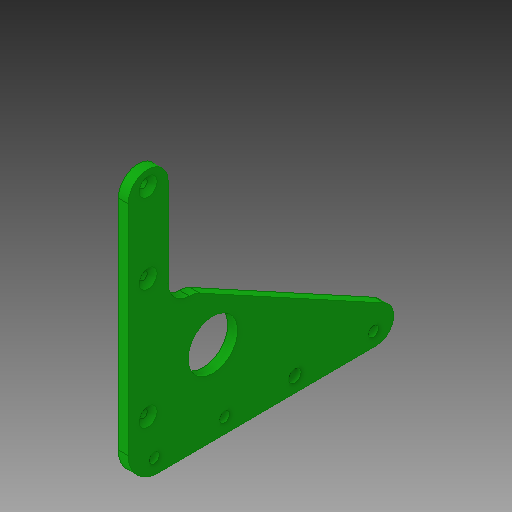
# Autodesk Inventor part: support plate
Saved by Autodesk Inventor 2017 SP1 (Build 210196100, 196)
## iProperties
Created: 2018-01-20
Part Number: support plate
Material: Aluminum 6061
Document SubType Name: Modeling
Designer: Ben
Density: 2.7 g/cm^3
Appearance: Dark Green
Mass: 193.553 g
Surface Area: 279.348 cm^2
Volume: 71.6862 cm^3
Author: Ben
Autodesk Inventor part; units mm, degrees
ref_plane "YZ Plane" through (0, 0, 0) normal (1, 0, 0) x (0, 1, 0)
ref_plane "XZ Plane" through (0, 0, 0) normal (0, 1, 0) x (-1, 0, 0)
ref_plane "XY Plane" through (0, 0, 0) normal (0, 0, 1) x (1, 0, 0)
sketch "Sketch1" plane through (0, 0, 0) normal (1, 0, 0) x (0, 1, 0)
  circle A0 centre (0, 0) radius 2.667
  circle A1 centre (76.2, 0) radius 2.667
  circle A2 centre (127, 0) radius 2.667
  line L0 (127, 0) -> (0, 0) construction
  line L1 (-15.2262, 12.7) -> (123.825, 12.7)
  line L2 (123.825, -12.7) -> (67.056, -12.7)
  line L3 (-33.4867, -145.5769) -> (-34.2759, -6.4581)
  line L4 (-12.7, -150.8212) -> (-12.7, 0) construction
  line L5 (-12.7, 0) -> (0, 0) construction
  line L6 (136.525, 0) -> (127, 0) construction
  circle A3 centre (-24.765, -3.937) radius 3.302
  circle A4 centre (-24.511, -48.7165) radius 3.302
  circle A5 centre (-24.257, -93.496) radius 4.064
  line L7 (-24.257, -93.496) -> (-24.511, -48.7165) construction
  line L8 (-24.511, -48.7165) -> (-24.765, -3.937) construction
  arc A6 (123.825, -12.7) -> (123.825, 12.7) centre (123.825, 0) ccw
  arc A7 (-15.2262, 12.7) -> (-34.2759, -6.4581) centre (-15.2262, -6.35) ccw
  arc A8 (-33.4867, -145.5769) -> (-12.7, -150.8212) centre (-22.416, -145.5141) ccw
  arc A9 (67.056, -12.7) -> (53.34, -26.416) centre (67.056, -26.416) ccw
  arc A10 (51.6613, -32.991) -> (53.34, -26.416) centre (39.624, -26.416) ccw
  line L9 (-12.7, -150.8212) -> (51.6613, -32.991)
  circle A11 centre (-24.765, -143.633) radius 3.302
  line L10 (-24.765, -143.633) -> (-24.257, -93.496) construction
  line L11 (-24.765, -143.633) -> (-24.765, -156.333) construction
  circle A12 centre (19.05, -41.275) radius 15.875
  circle A13 centre (19.05, -41.275) radius 12.7 construction
  line L12 (19.05, -28.575) -> (148.2391, -28.575) construction
  line L13 (53.34, 0) -> (53.34, -26.416) construction
  dimension "d34" = 25.4
  dimension "d0" = 5.334
  dimension "d1" = 127
  dimension "d3" = 12.7
  dimension "d7" = 6.604
  dimension "d9" = 3.937
  dimension "d10" = 44.7802
  dimension "d13" = 25.4
  dimension "d14" = 9.525
  dimension "d15" = 19.05
  dimension "d16" = 9.525
  dimension "d20" = 13.716
  dimension "d21" = 13.716
  dimension "d24" = 50.1396
  dimension "d25" = 12.065
  dimension "d26" = 11.557
  dimension "d27" = 12.065
  dimension "d28" = 8.128
  dimension "d29" = 12.7
  dimension "d33" = 31.75
  dimension "d35" = 31.75
  dimension "d37" = 76.2
  dimension "d38" = 66.04
  dimension "d39" = 28.575
  constraints: 28 end point, 13 centre point, 12 point on circle, 9 tangent, 5 equal radius, 4 horizontal, 3 collinear, 3 point on line, 3 vertical, 2 coincident, 1 perpendicular, 1 vertical alignment, 2 other
  measures "d0" diameter of A0
  measures "d1" distance of L0.start L0.end
  measures "d3" distance from line of point (0, 0) L4
  measures "d7" diameter of A3
  measures "d9" vertical distance of L8.end point (0, 0)
  measures "d10" distance of L7.end L8.end
  measures "d13" distance between parallel lines of L1 L2
  measures "d14" distance of L6.start L0.start
  measures "d15" radius of A7
  measures "d16" distance between parallel lines of L7 L3
  measures "d20" radius of A9
  measures "d21" radius of A10
  measures "d24" distance of L7.start L10.start
  measures "d25" distance from line of L4 L8.end
  measures "d26" distance from line of L4 L7.start
  measures "d27" distance from line of L4 L10.start
  measures "d28" diameter of A5
  measures "d29" distance of L10.start L11.end
  measures "d33" diameter of A12
  measures "d35" distance from line of L4 A12.centre
  measures "d37" distance of point (0, 0) A1.centre
  measures "d38" distance between parallel lines of L4 L13
  measures "d39" distance between parallel lines of L0 L12
extrude "Extrusion1" add sketch "Sketch1" along normal mid plane 6.35
chamfer "Chamfer1" distance 3.175 angle 45 3 edges at (3.175, 124.333, 0) (3.175, 73.533, 0) (3.175, -2.667, 0)
equation "\"d21\" = d20"
body "Solid1"
